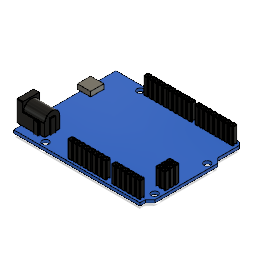
arduinoLeonardo (Autodesk Fusion 360 design; units mm, degrees)
Autodesk Fusion 360 part; units mm, degrees
note: some values were not read from the file. Chosen so that the rebuilt part matches the saved one: a direction; which face or edge a step refers to.
sketch "Sketch1" plane through (0, 0, 0) normal (0, 1, 0) x (1, 0, 0) in component "PCB"
  line L0 (0, 0) -> (64.5524, 0)
  line L1 (66.2, -1.6476) -> (66.2, -13)
  line L2 (66.2, -53.6) -> (0, -53.6)
  line L3 (0, -53.6) -> (0, 0)
  line L4 (64.5524, 0) -> (66.2, -1.6476)
  line L5 (64.5524, 0) -> (68.3345, 0) construction
  line L6 (64.5524, 0) -> (66.2, 0) construction
  line L7 (66.2, -13) -> (66.2, -50.8) construction
  line L8 (66.2, 0) -> (66.2, -1.6476) construction
  line L9 (66.2, -31.4728) -> (68.7, -31.4728) construction
  line L10 (66.2, -50.8) -> (66.2, -53.6)
  line L11 (66.2, -50.8) -> (68.7, -48.3)
  line L12 (66.2, -50.8) -> (70.1598, -50.8) construction
  line L13 (66.2, -13) -> (68.7, -15.5)
  line L14 (66.2, -13) -> (69.983, -13) construction
  line L15 (68.7, -15.5) -> (68.7, -48.3)
  dimension "d1" = 66.2
  dimension "d2" = 53.6
  dimension "d3" = 45
  dimension "d4" = 2.33
  dimension "d5" = 13
  dimension "d6" = 2.5
  dimension "d7" = 2.8
  dimension "d8" = 45
  dimension "d9" = 45
  dimension "d42" = 0
  dimension "d43" = 0
  dimension "d44" = 0
  dimension "d45" = 0
  dimension "d178" = 0
  dimension "d179" = 0
  dimension "d180" = 0
  dimension "d181" = 0
  measures "d3" angle of L4 L5
  measures "d8" angle of L11 L12
  measures "d9" angle of L13 L14
extrude "Extrude1" add sketch "Sketch1" along normal blind 1.62 makes body 1 in component "PCB"
sketch "Sketch1 (1)" plane through (0, 1.62, 0) normal (0, 1, 0) x (-1, 0, 0) in component "PCB"
  line L0 (-66.2, 50.8) -> (-68.7, 48.3)
  line L1 (-68.7, 48.3) -> (-68.7, 15.5)
  line L2 (-68.7, 15.5) -> (-66.2, 13)
  line L3 (-66.2, 13) -> (-66.2, 1.6476)
  line L4 (-66.2, 1.6476) -> (-64.5524, 0)
  line L5 (-64.5524, 0) -> (0, 0)
  line L6 (0, 0) -> (0, 53.6)
  line L7 (0, 53.6) -> (-66.2, 53.6)
  line L8 (-66.2, 53.6) -> (-66.2, 50.8)
  line L9 (-68.7, 31.9) -> (-67.7, 31.9) construction
  line L10 (-67.7, 18.15) -> (-67.7, 45.65) construction
  line L11 (-67.7, 18.15) -> (-65.95, 18.15) construction
  line L12 (-67.7, 45.65) -> (-65.95, 45.65) construction
  line L13 (-14, 53.6) -> (-14, 52.6) construction
  line L14 (-15.5, 0) -> (-15.5, 1) construction
  line L15 (-15.5, 1) -> (-15.5, 2.75) construction
  line L16 (-14, 52.6) -> (-14, 50.85) construction
  line L17 (0, 2.75) -> (-15.5, 2.75) construction
  line L18 (0, 50.85) -> (-14, 50.85) construction
  dimension "d12" = 1
  dimension "d13" = 27.5
  dimension "d14" = 1.75
  dimension "d15" = 1
  dimension "d16" = 1
  dimension "d17" = 1.75
  dimension "d18" = 1.75
  dimension "d19" = 15.5
  dimension "d20" = 14
  measures "d13" distance of L5.end
  measures "d20" distance of L5.end
hole "Hole1" at (15.5, 1.62, 2.75) at (14, 1.62, 50.85) at (65.95, 1.62, 45.65) at (65.95, 1.62, 18.15) direction (0, -1, 0) diameter 3.5 depth 1.62 tip angle 118 bodies 1 in component "PCB"
sketch "Sketch2" plane through (0, 1.62, 0) normal (0, 1, 0) x (-1, 0, 0) in component "PCB"
  circle A0 centre (-65.95, 45.65) radius 1.75
  circle A1 centre (-15.5, 2.75) radius 1.75
  circle A2 centre (-14, 50.85) radius 1.75
  circle A3 centre (-65.95, 18.15) radius 1.75
  line L0 (-66.2, 50.8) -> (-68.7, 48.3)
  line L1 (-68.7, 48.3) -> (-68.7, 15.5)
  line L2 (-68.7, 15.5) -> (-66.2, 13)
  line L3 (-66.2, 13) -> (-66.2, 1.6476)
  line L4 (-66.2, 1.6476) -> (-64.5524, 0)
  line L5 (-64.5524, 0) -> (0, 0)
  line L6 (0, 0) -> (0, 53.6)
  line L7 (0, 53.6) -> (-66.2, 53.6)
  line L8 (-66.2, 53.6) -> (-66.2, 50.8)
  line L9 (-64.3788, 0) -> (-64.3788, 2.5) construction
  line L10 (-65.4815, 53.6) -> (-65.4815, 51.1) construction
  line L11 (-66.2, 2.5) -> (-63.7, 2.5) construction
  line L12 (-66.2, 51.1) -> (-63.7, 51.1) construction
  line L13 (-63.7, 51.1) -> (-61.16, 51.1) construction
  line L14 (-61.16, 51.1) -> (-58.62, 51.1) construction
  line L15 (-58.62, 51.1) -> (-56.08, 51.1) construction
  line L16 (-56.08, 51.1) -> (-53.54, 51.1) construction
  line L17 (-53.54, 51.1) -> (-51, 51.1) construction
  line L18 (-51, 51.1) -> (-46, 51.1) construction
  line L19 (-46, 51.1) -> (-43.46, 51.1) construction
  line L20 (-43.46, 51.1) -> (-40.92, 51.1) construction
  line L21 (-40.92, 51.1) -> (-38.38, 51.1) construction
  line L22 (-38.38, 51.1) -> (-35.84, 51.1) construction
  line L23 (-35.84, 51.1) -> (-33.3, 51.1) construction
  line L24 (-33.3, 51.1) -> (-30.76, 51.1) construction
  line L25 (-30.76, 51.1) -> (-28.22, 51.1) construction
  line L26 (-28.22, 51.1) -> (-25.68, 51.1) construction
  line L27 (-63.7, 2.5) -> (-61.16, 2.5) construction
  line L28 (-61.16, 2.5) -> (-58.62, 2.5) construction
  line L29 (-58.62, 2.5) -> (-56.08, 2.5) construction
  line L30 (-56.08, 2.5) -> (-53.54, 2.5) construction
  line L31 (-53.54, 2.5) -> (-51, 2.5) construction
  line L32 (-51, 2.5) -> (-48.46, 2.5) construction
  line L33 (-45.92, 2.5114) -> (-48.46, 2.5) construction
  line L34 (-45.92, 2.5114) -> (-42.1201, 2.5284) construction
  line L35 (-42.1201, 2.5284) -> (-39.5801, 2.5398) construction
  line L36 (-39.5801, 2.5398) -> (-37.0401, 2.5511) construction
  line L37 (-37.0401, 2.5511) -> (-34.5001, 2.5625) construction
  line L38 (-34.5001, 2.5625) -> (-31.9602, 2.5739) construction
  line L39 (-31.9602, 2.5739) -> (-29.4202, 2.5853) construction
  line L40 (-29.4202, 2.5853) -> (-26.8802, 2.5966) construction
  line L41 (-26.8802, 2.5966) -> (-24.3402, 2.608) construction
  line L42 (-24.3402, 2.608) -> (-21.8003, 2.6194) construction
  line L43 (-21.8003, 2.6194) -> (-19.2603, 2.6307) construction
  line L44 (-68.7, 40.6001) -> (-66.2, 40.6001) construction
  line L45 (-65.9335, 43.9001) -> (-65.9335, 40.6001) construction
  line L46 (-66.2, 40.6001) -> (-66.2, 38.0601) construction
  line L47 (-66.2, 38.0601) -> (-66.2, 35.5201) construction
  line L48 (-66.2, 35.5201) -> (-63.66, 35.5201) construction
  line L49 (-63.66, 35.5201) -> (-63.66, 38.0601) construction
  line L50 (-63.66, 38.0601) -> (-63.66, 40.6001) construction
  dimension "d24" = 2.5
  dimension "d25" = 2.5
  dimension "d26" = 2.5
  dimension "d27" = 2.5
  dimension "d28" = 2.54
  dimension "d29" = 5
  dimension "d30" = 2.54
  dimension "d31" = 3.8
  dimension "d32" = 2.5
  dimension "d33" = 3.3
  dimension "d34" = 2.54
  measures "d24" distance of L5.end
hole "Hole2" at (63.7, 1.62, 51.1) at (61.16, 1.62, 51.1) at (58.62, 1.62, 51.1) at (56.08, 1.62, 51.1) at (53.54, 1.62, 51.1) at (51, 1.62, 51.1) at (46, 1.62, 51.1) at (43.46, 1.62, 51.1) at (40.92, 1.62, 51.1) at (38.38, 1.62, 51.1) at (35.84, 1.62, 51.1) at (33.3, 1.62, 51.1) at (30.76, 1.62, 51.1) at (28.22, 1.62, 51.1) at (63.66, 1.62, 40.6001) at (63.66, 1.62, 38.0601) at (63.66, 1.62, 35.5201) at (66.2, 1.62, 35.5201) at (66.2, 1.62, 38.0601) at (66.2, 1.62, 40.6001) at (63.7, 1.62, 2.5) at (61.16, 1.62, 2.5) at (58.62, 1.62, 2.5) at (56.08, 1.62, 2.5) at (53.54, 1.62, 2.5) at (51, 1.62, 2.5) at (48.46, 1.62, 2.5) at (45.92, 1.62, 2.5114) at (42.1201, 1.62, 2.5284) at (39.5801, 1.62, 2.5398) at (37.0401, 1.62, 2.5511) at (34.5001, 1.62, 2.5625) at (31.9602, 1.62, 2.5739) at (29.4202, 1.62, 2.5853) at (26.8802, 1.62, 2.5966) at (24.3402, 1.62, 2.608) at (21.8003, 1.62, 2.6194) at (19.2603, 1.62, 2.6307) direction (0, -1, 0) diameter 0.635 depth 1.62 tip angle 118 bodies 1 in component "PCB"
sketch "Sketch1 (2)" plane through (0, 0, 0) normal (0, 1, 0) x (1, 0, 0) in component "Pin"
  line L0 (0, 0) -> (5.08, 0)
  line L1 (5.08, 0) -> (5.08, -0.635)
  line L2 (5.08, -0.635) -> (0, -0.635)
  line L3 (0, -0.635) -> (0, 0)
  dimension "d2_1" = 0.635
  dimension "d3_1" = 5.08
  measures "d3_1" distance of L0.start
extrude "Extrude1'" add sketch "Sketch1 (2)" along normal blind 0.635 separate body makes body 2 in component "Pin"
chamfer "Chamfer1" distance 0.1905 angle 45 4 edges at (0, 0.3175, 0.635) (0, 0.635, 0.3175) (0, 0.3175, 0) (0, 0, 0.3175) on bodies 2 in component "Pin"
sketch "Sketch1 (3)" plane through (0, 0, 0) normal (0, 1, 0) x (1, 0, 0) in component "Plastic"
  line L0 (0, -0.3175) -> (3.81, -0.3175)
  line L1 (3.81, -1.0795) -> (3.81, 0.4445)
  line L2 (3.81, 0.4445) -> (3.8102, 0.9525) construction
  line L3 (3.81, -1.0795) -> (3.81, -1.5875) construction
  line L4 (3.81, 0.4445) -> (3.175, 0.4445)
  line L5 (3.81, -1.0795) -> (3.175, -1.0795)
  line L6 (3.175, -1.0795) -> (3.175, -1.5875)
  line L7 (3.175, 0.4445) -> (3.175, 0.9525)
  line L8 (3.175, 0.9525) -> (11.811, 0.9525)
  line L9 (11.811, 0.9525) -> (11.811, -1.5875)
  line L10 (3.175, -1.5875) -> (11.811, -1.5875)
  line L11 (0, -0.1905) -> (0, -0.4445)
  dimension "d7_1" = 3.81
  dimension "d8_1" = 1.524
  dimension "d9_1" = 0.508
  dimension "d11_1" = 0.635
  dimension "d12_1" = 8.636
  measures "d7_1" distance of origin
extrude "Extrude1''" add sketch "Sketch1 (3)" along normal mid plane 2.54 from surface at 0.3175 separate body makes body 3 in component "Plastic"
chamfer "Chamfer1'" distance 0.4 angle 45 4 edges at (7.493, 1.5875, -0.9525) (7.493, -0.9525, -0.9525) (7.493, 1.5875, 1.5875) (7.493, -0.9525, 1.5875) on bodies 3 in component "Plastic"
sketch "Sketch1 (4)" plane through (0, 0, 0) normal (0, 0, 1) x (1, 0, 0) in component "Pins straight female v5"
  line L0 (0, 0.1905) -> (0, 0.4445)
  line L1 (0, 0.3175) -> (0, 14)
other "PathPattern1" in component "Header"
sketch "Sketch1 (1) (2)" plane through (11.811, 0, 0) normal (1, 0, 0) x (0, 0, -1) in component "Plastic"
  line L0 (-1.5875, -0.5525) -> (-1.1875, -0.9525)
  line L1 (-1.1875, -0.9525) -> (0.5525, -0.9525)
  line L2 (0.5525, -0.9525) -> (0.9525, -0.5525)
  line L3 (0.9525, -0.5525) -> (0.9525, 1.1875)
  line L4 (0.9525, 1.1875) -> (0.5525, 1.5875)
  line L5 (0.5525, 1.5875) -> (-1.1875, 1.5875)
  line L6 (-1.1875, 1.5875) -> (-1.5875, 1.1875)
  line L7 (-1.5875, 1.1875) -> (-1.5875, -0.5525)
  line L8 (0.9525, 0.3175) -> (-0.3175, 0.3175) construction
  line L9 (-0.3175, 1.5875) -> (-0.3175, 0.3175) construction
  line L10 (-0.3175, 0.635) -> (0, 0.635)
  line L11 (0, 0.3175) -> (0, 0)
  line L12 (0, 0) -> (-0.635, 0)
  line L13 (-0.635, 0) -> (-0.635, 0.635)
  line L14 (0, 0.635) -> (0, 0.3175)
  line L15 (-0.635, 0.635) -> (-0.3175, 0.635)
  dimension "d24_1" = 0.635
  dimension "d25_1" = 0.635
  measures "d25_1" distance of L11.end
extrude "Extrude1'''" cut sketch "Sketch1 (1) (2)" against normal blind 5.5 contours L10 L11 L12 L13 L14 L15 bodies 3 in component "Plastic"
chamfer "Chamfer1''" distance 0.6 angle 45 4 edges at (11.811, 0, 0.3175) (11.811, 0.3175, 0) (11.811, 0.635, 0.3175) (11.811, 0.3175, 0.635) on bodies 3 in component "Plastic"
sketch "Sketch1 (5)" plane through (0, 0, 0) normal (0, 1, 0) x (1, 0, 0) in component "Pin (1)"
  line L0 (0, 0) -> (5.08, 0)
  line L1 (5.08, 0) -> (5.08, -0.635)
  line L2 (5.08, -0.635) -> (0, -0.635)
  line L3 (0, -0.635) -> (0, 0)
  dimension "d2_2" = 0.635
  dimension "d3_2" = 5.08
  measures "d3_2" distance of L0.start
extrude "Extrude1''''" add sketch "Sketch1 (5)" along normal blind 0.635 separate body makes body 4 in component "Pin (1)"
chamfer "Chamfer1'''" distance 0.1905 angle 45 4 edges at (0, 0.3175, 0.635) (0, 0.635, 0.3175) (0, 0.3175, 0) (0, 0, 0.3175) on bodies 4 in component "Pin (1)"
sketch "Sketch1 (6)" plane through (0, 0, 0) normal (0, 1, 0) x (1, 0, 0) in component "Plastic (1)"
  line L0 (0, -0.3175) -> (3.81, -0.3175)
  line L1 (3.81, -1.0795) -> (3.81, 0.4445)
  line L2 (3.81, 0.4445) -> (3.8102, 0.9525) construction
  line L3 (3.81, -1.0795) -> (3.81, -1.5875) construction
  line L4 (3.81, 0.4445) -> (3.175, 0.4445)
  line L5 (3.81, -1.0795) -> (3.175, -1.0795)
  line L6 (3.175, -1.0795) -> (3.175, -1.5875)
  line L7 (3.175, 0.4445) -> (3.175, 0.9525)
  line L8 (3.175, 0.9525) -> (11.811, 0.9525)
  line L9 (11.811, 0.9525) -> (11.811, -1.5875)
  line L10 (3.175, -1.5875) -> (11.811, -1.5875)
  line L11 (0, -0.1905) -> (0, -0.4445)
  dimension "d7_2" = 3.81
  dimension "d8_2" = 1.524
  dimension "d9_2" = 0.508
  dimension "d11_2" = 0.635
  dimension "d12_2" = 8.636
  measures "d7_2" distance of origin
extrude "Extrude1'''''" add sketch "Sketch1 (6)" along normal mid plane 2.54 from surface at 0.3175 separate body makes body 5 in component "Plastic (1)"
chamfer "Chamfer1''''" distance 0.4 angle 45 4 edges at (7.493, 1.5875, -0.9525) (7.493, -0.9525, -0.9525) (7.493, 1.5875, 1.5875) (7.493, -0.9525, 1.5875) on bodies 5 in component "Plastic (1)"
sketch "Sketch1 (7)" plane through (0, 0, 0) normal (0, 0, 1) x (1, 0, 0) in component "Pins straight female v6"
  line L0 (0, 0.1905) -> (0, 0.4445)
  line L1 (0, 0.3175) -> (0, 14)
other "PathPattern1'" in component "Header (1)"
sketch "Sketch1 (1) (3)" plane through (11.811, 0, 0) normal (1, 0, 0) x (0, 0, -1) in component "Plastic (1)"
  line L0 (-1.5875, -0.5525) -> (-1.1875, -0.9525)
  line L1 (-1.1875, -0.9525) -> (0.5525, -0.9525)
  line L2 (0.5525, -0.9525) -> (0.9525, -0.5525)
  line L3 (0.9525, -0.5525) -> (0.9525, 1.1875)
  line L4 (0.9525, 1.1875) -> (0.5525, 1.5875)
  line L5 (0.5525, 1.5875) -> (-1.1875, 1.5875)
  line L6 (-1.1875, 1.5875) -> (-1.5875, 1.1875)
  line L7 (-1.5875, 1.1875) -> (-1.5875, -0.5525)
  line L8 (0.9525, 0.3175) -> (-0.3175, 0.3175) construction
  line L9 (-0.3175, 1.5875) -> (-0.3175, 0.3175) construction
  line L10 (-0.3175, 0.635) -> (0, 0.635)
  line L11 (0, 0.3175) -> (0, 0)
  line L12 (0, 0) -> (-0.635, 0)
  line L13 (-0.635, 0) -> (-0.635, 0.635)
  line L14 (0, 0.635) -> (0, 0.3175)
  line L15 (-0.635, 0.635) -> (-0.3175, 0.635)
  dimension "d24_2" = 0.635
  dimension "d25_2" = 0.635
  measures "d25_2" distance of L11.end
extrude "Extrude1''''''" cut sketch "Sketch1 (1) (3)" against normal blind 5.5 contours L10 L11 L12 L13 L14 L15 bodies 5 in component "Plastic (1)"
chamfer "Chamfer1'''''" distance 0.6 angle 45 4 edges at (11.811, 0, 0.3175) (11.811, 0.3175, 0) (11.811, 0.635, 0.3175) (11.811, 0.3175, 0.635) on bodies 5 in component "Plastic (1)"
sketch "Sketch1 (8)" plane through (0, 0, 0) normal (0, 1, 0) x (1, 0, 0) in component "Pin (2)"
  line L0 (0, 0) -> (5.08, 0)
  line L1 (5.08, 0) -> (5.08, -0.635)
  line L2 (5.08, -0.635) -> (0, -0.635)
  line L3 (0, -0.635) -> (0, 0)
  dimension "d2_3" = 0.635
  dimension "d3_3" = 5.08
  dimension "d38" = 0
  dimension "d39" = 0
  dimension "d40" = 0
  dimension "d41" = 0
  measures "d3_3" distance of L0.start
extrude "Extrude1'''''''" add sketch "Sketch1 (8)" along normal blind 0.635 separate body makes body 6 in component "Pin (2)"
chamfer "Chamfer1''''''" distance 0.1905 angle 45 4 edges at (0, 0.3175, 0.635) (0, 0.635, 0.3175) (0, 0.3175, 0) (0, 0, 0.3175) on bodies 6 in component "Pin (2)"
sketch "Sketch1 (9)" plane through (0, 0, 0) normal (0, 1, 0) x (1, 0, 0) in component "Plastic (2)"
  line L0 (0, -0.3175) -> (3.81, -0.3175)
  line L1 (3.81, -1.0795) -> (3.81, 0.4445)
  line L2 (3.81, 0.4445) -> (3.8102, 0.9525) construction
  line L3 (3.81, -1.0795) -> (3.81, -1.5875) construction
  line L4 (3.81, 0.4445) -> (3.175, 0.4445)
  line L5 (3.81, -1.0795) -> (3.175, -1.0795)
  line L6 (3.175, -1.0795) -> (3.175, -1.5875)
  line L7 (3.175, 0.4445) -> (3.175, 0.9525)
  line L8 (3.175, 0.9525) -> (11.811, 0.9525)
  line L9 (11.811, 0.9525) -> (11.811, -1.5875)
  line L10 (3.175, -1.5875) -> (11.811, -1.5875)
  line L11 (0, -0.1905) -> (0, -0.4445)
  dimension "d7_3" = 3.81
  dimension "d8_3" = 1.524
  dimension "d9_3" = 0.508
  dimension "d11_3" = 0.635
  dimension "d12_3" = 8.636
  measures "d7_3" distance of origin
extrude "Extrude1''''''''" add sketch "Sketch1 (9)" along normal mid plane 2.54 from surface at 0.3175 separate body makes body 7 in component "Plastic (2)"
chamfer "Chamfer1'''''''" distance 0.4 angle 45 4 edges at (7.493, 1.5875, -0.9525) (7.493, -0.9525, -0.9525) (7.493, 1.5875, 1.5875) (7.493, -0.9525, 1.5875) on bodies 7 in component "Plastic (2)"
sketch "Sketch1 (10)" plane through (0, 0, 0) normal (0, 0, 1) x (1, 0, 0) in component "Pins straight female v7"
  line L0 (0, 0.1905) -> (0, 0.4445)
  line L1 (0, 0.3175) -> (0, 14)
other "PathPattern1''" in component "Header (2)"
sketch "Sketch1 (1) (4)" plane through (11.811, 0, 0) normal (1, 0, 0) x (0, 0, -1) in component "Plastic (2)"
  line L0 (-1.5875, -0.5525) -> (-1.1875, -0.9525)
  line L1 (-1.1875, -0.9525) -> (0.5525, -0.9525)
  line L2 (0.5525, -0.9525) -> (0.9525, -0.5525)
  line L3 (0.9525, -0.5525) -> (0.9525, 1.1875)
  line L4 (0.9525, 1.1875) -> (0.5525, 1.5875)
  line L5 (0.5525, 1.5875) -> (-1.1875, 1.5875)
  line L6 (-1.1875, 1.5875) -> (-1.5875, 1.1875)
  line L7 (-1.5875, 1.1875) -> (-1.5875, -0.5525)
  line L8 (0.9525, 0.3175) -> (-0.3175, 0.3175) construction
  line L9 (-0.3175, 1.5875) -> (-0.3175, 0.3175) construction
  line L10 (-0.3175, 0.635) -> (0, 0.635)
  line L11 (0, 0.3175) -> (0, 0)
  line L12 (0, 0) -> (-0.635, 0)
  line L13 (-0.635, 0) -> (-0.635, 0.635)
  line L14 (0, 0.635) -> (0, 0.3175)
  line L15 (-0.635, 0.635) -> (-0.3175, 0.635)
  dimension "d24_3" = 0.635
  dimension "d25_3" = 0.635
  measures "d25_3" distance of L11.end
extrude "Extrude1'''''''''" cut sketch "Sketch1 (1) (4)" against normal blind 5.5 contours L10 L11 L12 L13 L14 L15 bodies 7 in component "Plastic (2)"
chamfer "Chamfer1''''''''" distance 0.6 angle 45 4 edges at (11.811, 0, 0.3175) (11.811, 0.3175, 0) (11.811, 0.635, 0.3175) (11.811, 0.3175, 0.635) on bodies 7 in component "Plastic (2)"
sketch "Sketch1 (11)" plane through (0, 0, 0) normal (0, 1, 0) x (1, 0, 0) in component "Pin (3)"
  line L0 (0, 0) -> (5.08, 0)
  line L1 (5.08, 0) -> (5.08, -0.635)
  line L2 (5.08, -0.635) -> (0, -0.635)
  line L3 (0, -0.635) -> (0, 0)
  dimension "d2_4" = 0.635
  dimension "d3_4" = 5.08
  measures "d3_4" distance of L0.start
extrude "Extrude1''''''''''" add sketch "Sketch1 (11)" along normal blind 0.635 separate body makes body 8 in component "Pin (3)"
chamfer "Chamfer1'''''''''" distance 0.1905 angle 45 4 edges at (0, 0.3175, 0.635) (0, 0.635, 0.3175) (0, 0.3175, 0) (0, 0, 0.3175) on bodies 8 in component "Pin (3)"
sketch "Sketch1 (12)" plane through (0, 0, 0) normal (0, 1, 0) x (1, 0, 0) in component "Plastic (3)"
  line L0 (0, -0.3175) -> (3.81, -0.3175)
  line L1 (3.81, -1.0795) -> (3.81, 0.4445)
  line L2 (3.81, 0.4445) -> (3.8102, 0.9525) construction
  line L3 (3.81, -1.0795) -> (3.81, -1.5875) construction
  line L4 (3.81, 0.4445) -> (3.175, 0.4445)
  line L5 (3.81, -1.0795) -> (3.175, -1.0795)
  line L6 (3.175, -1.0795) -> (3.175, -1.5875)
  line L7 (3.175, 0.4445) -> (3.175, 0.9525)
  line L8 (3.175, 0.9525) -> (11.811, 0.9525)
  line L9 (11.811, 0.9525) -> (11.811, -1.5875)
  line L10 (3.175, -1.5875) -> (11.811, -1.5875)
  line L11 (0, -0.1905) -> (0, -0.4445)
  dimension "d7_4" = 3.81
  dimension "d8_4" = 1.524
  dimension "d9_4" = 0.508
  dimension "d11_4" = 0.635
  dimension "d12_4" = 8.636
  measures "d7_4" distance of origin
extrude "Extrude1'''''''''''" add sketch "Sketch1 (12)" along normal mid plane 2.54 from surface at 0.3175 separate body makes body 9 in component "Plastic (3)"
chamfer "Chamfer1''''''''''" distance 0.4 angle 45 4 edges at (7.493, 1.5875, -0.9525) (7.493, -0.9525, -0.9525) (7.493, 1.5875, 1.5875) (7.493, -0.9525, 1.5875) on bodies 9 in component "Plastic (3)"
sketch "Sketch1 (13)" plane through (0, 0, 0) normal (0, 0, 1) x (1, 0, 0) in component "Pins straight female v8"
  line L0 (0, 0.1905) -> (0, 0.4445)
  line L1 (0, 0.3175) -> (0, 14)
other "PathPattern1'''" in component "Header (3)"
sketch "Sketch1 (1) (5)" plane through (11.811, 0, 0) normal (1, 0, 0) x (0, 0, -1) in component "Plastic (3)"
  line L0 (-1.5875, -0.5525) -> (-1.1875, -0.9525)
  line L1 (-1.1875, -0.9525) -> (0.5525, -0.9525)
  line L2 (0.5525, -0.9525) -> (0.9525, -0.5525)
  line L3 (0.9525, -0.5525) -> (0.9525, 1.1875)
  line L4 (0.9525, 1.1875) -> (0.5525, 1.5875)
  line L5 (0.5525, 1.5875) -> (-1.1875, 1.5875)
  line L6 (-1.1875, 1.5875) -> (-1.5875, 1.1875)
  line L7 (-1.5875, 1.1875) -> (-1.5875, -0.5525)
  line L8 (0.9525, 0.3175) -> (-0.3175, 0.3175) construction
  line L9 (-0.3175, 1.5875) -> (-0.3175, 0.3175) construction
  line L10 (-0.3175, 0.635) -> (0, 0.635)
  line L11 (0, 0.3175) -> (0, 0)
  line L12 (0, 0) -> (-0.635, 0)
  line L13 (-0.635, 0) -> (-0.635, 0.635)
  line L14 (0, 0.635) -> (0, 0.3175)
  line L15 (-0.635, 0.635) -> (-0.3175, 0.635)
  dimension "d24_4" = 0.635
  dimension "d25_4" = 0.635
  measures "d25_4" distance of L11.end
extrude "Extrude1''''''''''''" cut sketch "Sketch1 (1) (5)" against normal blind 5.5 contours L10 L11 L12 L13 L14 L15 bodies 9 in component "Plastic (3)"
chamfer "Chamfer1'''''''''''" distance 0.6 angle 45 4 edges at (11.811, 0, 0.3175) (11.811, 0.3175, 0) (11.811, 0.635, 0.3175) (11.811, 0.3175, 0.635) on bodies 9 in component "Plastic (3)"
sketch "Sketch3" plane through (0, 1.62, 0) normal (0, 1, 0) x (-1, 0, 0) in component "PCB"
  circle A0 centre (-21.8003, 2.6194) radius 0.3175
  circle A1 centre (-26.8802, 2.5966) radius 0.3175
  circle A2 centre (-31.9602, 2.5739) radius 0.3175
  circle A3 centre (-37.0401, 2.5511) radius 0.3175
  circle A4 centre (-42.1201, 2.5284) radius 0.3175
  circle A5 centre (-48.46, 2.5) radius 0.3175
  circle A6 centre (-53.54, 2.5) radius 0.3175
  circle A7 centre (-58.62, 2.5) radius 0.3175
  circle A8 centre (-63.7, 2.5) radius 0.3175
  circle A9 centre (-66.2, 38.0601) radius 0.3175
  circle A10 centre (-63.66, 35.5201) radius 0.3175
  circle A11 centre (-63.66, 40.6001) radius 0.3175
  circle A12 centre (-30.76, 51.1) radius 0.3175
  circle A13 centre (-35.84, 51.1) radius 0.3175
  circle A14 centre (-40.92, 51.1) radius 0.3175
  circle A15 centre (-46, 51.1) radius 0.3175
  circle A16 centre (-53.54, 51.1) radius 0.3175
  circle A17 centre (-58.62, 51.1) radius 0.3175
  circle A18 centre (-63.7, 51.1) radius 0.3175
  circle A19 centre (-61.16, 51.1) radius 0.3175
  circle A20 centre (-56.08, 51.1) radius 0.3175
  circle A21 centre (-51, 51.1) radius 0.3175
  circle A22 centre (-43.46, 51.1) radius 0.3175
  circle A23 centre (-38.38, 51.1) radius 0.3175
  circle A24 centre (-33.3, 51.1) radius 0.3175
  circle A25 centre (-28.22, 51.1) radius 0.3175
  circle A26 centre (-63.66, 38.0601) radius 0.3175
  circle A27 centre (-66.2, 35.5201) radius 0.3175
  circle A28 centre (-66.2, 40.6001) radius 0.3175
  circle A29 centre (-61.16, 2.5) radius 0.3175
  circle A30 centre (-56.08, 2.5) radius 0.3175
  circle A31 centre (-51, 2.5) radius 0.3175
  circle A32 centre (-45.92, 2.5114) radius 0.3175
  circle A33 centre (-39.5801, 2.5398) radius 0.3175
  circle A34 centre (-34.5001, 2.5625) radius 0.3175
  circle A35 centre (-29.4202, 2.5853) radius 0.3175
  circle A36 centre (-24.3402, 2.608) radius 0.3175
  circle A37 centre (-19.2603, 2.6307) radius 0.3175
  circle A38 centre (-65.95, 45.65) radius 1.75
  circle A39 centre (-15.5, 2.75) radius 1.75
  circle A40 centre (-14, 50.85) radius 1.75
  circle A41 centre (-65.95, 18.15) radius 1.75
  line L0 (-66.2, 50.8) -> (-68.7, 48.3)
  line L1 (-68.7, 48.3) -> (-68.7, 15.5)
  line L2 (-68.7, 15.5) -> (-66.2, 13)
  line L3 (-66.2, 13) -> (-66.2, 1.6476)
  line L4 (-66.2, 1.6476) -> (-64.5524, 0)
  line L5 (-64.5524, 0) -> (0, 0)
  line L6 (0, 0) -> (0, 53.6)
  line L7 (0, 53.6) -> (-66.2, 53.6)
  line L8 (-66.2, 53.6) -> (-66.2, 50.8)
  line L9 (-4, 0) -> (-4, 15) construction
  line L10 (0, 15) -> (-4, 15) construction
  line L11 (-4, 12.575) -> (-4, 17.425) construction
  dimension "d118" = 15
  dimension "d119" = 4
  dimension "d120" = 4.85
hole "Hole3" at (4, 1.62, 12.575) at (4, 1.62, 17.425) direction (0, -1, 0) diameter 0.635 depth 1.62 tip angle 118 bodies 1 in component "PCB"
sketch "Sketch1 (14)" plane through (0, 1.62, 0) normal (0, 1, 0) x (-1, 0, 0) in component "PCB"
  circle A0 centre (-4, 12.575) radius 0.3175
  circle A1 centre (-4, 17.425) radius 0.3175
  circle A2 centre (-21.8003, 2.6194) radius 0.3175
  circle A3 centre (-26.8802, 2.5966) radius 0.3175
  circle A4 centre (-31.9602, 2.5739) radius 0.3175
  circle A5 centre (-37.0401, 2.5511) radius 0.3175
  circle A6 centre (-42.1201, 2.5284) radius 0.3175
  circle A7 centre (-48.46, 2.5) radius 0.3175
  circle A8 centre (-53.54, 2.5) radius 0.3175
  circle A9 centre (-58.62, 2.5) radius 0.3175
  circle A10 centre (-63.7, 2.5) radius 0.3175
  circle A11 centre (-66.2, 38.0601) radius 0.3175
  circle A12 centre (-63.66, 35.5201) radius 0.3175
  circle A13 centre (-63.66, 40.6001) radius 0.3175
  circle A14 centre (-30.76, 51.1) radius 0.3175
  circle A15 centre (-35.84, 51.1) radius 0.3175
  circle A16 centre (-40.92, 51.1) radius 0.3175
  circle A17 centre (-46, 51.1) radius 0.3175
  circle A18 centre (-53.54, 51.1) radius 0.3175
  circle A19 centre (-58.62, 51.1) radius 0.3175
  circle A20 centre (-63.7, 51.1) radius 0.3175
  circle A21 centre (-61.16, 51.1) radius 0.3175
  circle A22 centre (-56.08, 51.1) radius 0.3175
  circle A23 centre (-51, 51.1) radius 0.3175
  circle A24 centre (-43.46, 51.1) radius 0.3175
  circle A25 centre (-38.38, 51.1) radius 0.3175
  circle A26 centre (-33.3, 51.1) radius 0.3175
  circle A27 centre (-28.22, 51.1) radius 0.3175
  circle A28 centre (-63.66, 38.0601) radius 0.3175
  circle A29 centre (-66.2, 35.5201) radius 0.3175
  circle A30 centre (-66.2, 40.6001) radius 0.3175
  circle A31 centre (-61.16, 2.5) radius 0.3175
  circle A32 centre (-56.08, 2.5) radius 0.3175
  circle A33 centre (-51, 2.5) radius 0.3175
  circle A34 centre (-45.92, 2.5114) radius 0.3175
  circle A35 centre (-39.5801, 2.5398) radius 0.3175
  circle A36 centre (-34.5001, 2.5625) radius 0.3175
  circle A37 centre (-29.4202, 2.5853) radius 0.3175
  circle A38 centre (-24.3402, 2.608) radius 0.3175
  circle A39 centre (-19.2603, 2.6307) radius 0.3175
  circle A40 centre (-65.95, 45.65) radius 1.75
  circle A41 centre (-15.5, 2.75) radius 1.75
  circle A42 centre (-14, 50.85) radius 1.75
  circle A43 centre (-65.95, 18.15) radius 1.75
  line L0 (-66.2, 50.8) -> (-68.7, 48.3)
  line L1 (-68.7, 48.3) -> (-68.7, 15.5)
  line L2 (-68.7, 15.5) -> (-66.2, 13)
  line L3 (-66.2, 13) -> (-66.2, 1.6476)
  line L4 (-66.2, 1.6476) -> (-64.5524, 0)
  line L5 (-64.5524, 0) -> (0, 0)
  line L6 (0, 0) -> (0, 53.6)
  line L7 (0, 53.6) -> (-66.2, 53.6)
  line L8 (-66.2, 53.6) -> (-66.2, 50.8)
  line L9 (0, 45.1) -> (-12, 45.1) construction
  line L10 (-12, 45.1) -> (-12, 53.6) construction
  dimension "d136" = 12
  dimension "d137" = 8.5
  measures "d136" distance of L5.end
sketch "Sketch1 (15)" plane through (0, 0, 0) normal (0, 1, 0) x (1, 0, 0) in component "DC Jack"
  line L0 (0, 0) -> (9, 0)
  line L1 (9, 0) -> (9, -11)
  line L2 (9, -11) -> (0, -11)
  line L3 (0, -11) -> (0, 0)
  dimension "d1_1" = 9
  dimension "d2_5" = 11
  measures "d1_1" distance of L0.start
  measures "d2_5" distance of L0.start
extrude "Extrude1'''''''''''''" add sketch "Sketch1 (15)" along normal blind 3.3 separate body makes body 10 in component "DC Jack"
sketch "Sketch2 (2)" plane through (0, 3.3, 0) normal (0, 1, 0) x (-1, 0, 0) in component "DC Jack"
  line L0 (0, 11) -> (-9, 11)
  line L1 (-9, 11) -> (-9, 0)
  line L2 (-9, 0) -> (0, 0)
  line L3 (0, 0) -> (0, 11)
  circle A0 centre (-4.5, 4.75) radius 3.95
  line L4 (-4.5, 0) -> (-4.5, 0.8) construction
  line L5 (-9, 4.75) -> (-8.45, 4.75)
  line L6 (0, 4.75) -> (-0.55, 4.75)
  dimension "d5_5" = 0.8
  dimension "d6_5" = 7.9
  measures "d6_5" diameter of A0
extrude "Extrude2" add sketch "Sketch2 (2)" along normal blind 8.5 contours L0 L1 L3 A0 L5 L6 | A0 bodies 10 in component "DC Jack"
sketch "Sketch3 (2)" plane through (0, 11.8, 0) normal (0, 1, 0) x (-1, 0, 0) in component "DC Jack"
  line L0 (0, 11) -> (-9, 11)
  line L1 (-9, 11) -> (-9, 4.75)
  line L2 (-9, 4.75) -> (-8.45, 4.75)
  arc A0 (-8.45, 4.75) -> (-0.55, 4.75) centre (-4.5, 4.75) ccw
  line L3 (-0.55, 4.75) -> (0, 4.75)
  line L4 (0, 4.75) -> (0, 11)
  line L5 (-0.55, 4.75) -> (-0.55, 11)
  line L6 (-8.45, 4.75) -> (-8.45, 11)
extrude "Extrude3" add sketch "Sketch3 (2)" along normal blind 2.4 contours L0 A0 L5 L6 bodies 10 in component "DC Jack"
sketch "Sketch4" plane through (0, 0, 0) normal (0, -1, 0) x (1, 0, 0) in component "DC Jack"
  line L0 (9, 11) -> (0, 11)
  line L1 (0, 11) -> (0, 0)
  line L2 (0, 0) -> (9, 0)
  line L3 (9, 0) -> (9, 11)
hole "Hole1'" at (4.5, 0, 4.75) direction (0, 1, 0) diameter 6.5 depth 9.6 tip angle 180 bodies 10 in component "DC Jack"
sketch "Sketch1 (16)" plane through (0, 9.6, 0) normal (0, -1, 0) x (1, 0, 0) in component "Connection"
  circle A0 centre (4.5, 4.75) radius 3.25
  circle A1 centre (4.5, 4.75) radius 1.25
  dimension "d14_5" = 2.5
  measures "d14_5" diameter of A1
extrude "Extrude1''''''''''''''" add sketch "Sketch1 (16)" along normal blind 8.1 separate body contours A1 makes body 11 in component "Connection"
ref_plane "WorkPlane1" through (1.2501, 0.7141, 4.7724) normal (0.999976, 0, -0.006903) x (0.006903, 0, 0.999976) in component "Connection"
ref_plane "WorkPlane2" through (3.2501, 2.383, 4.7654) normal (-0.999924, 0, 0.012358) x (0.012358, 0, 0.999924) in component "Connection"
ref_plane "WorkPlane3" through (2.2501, 2.383, 4.7764) normal (-0.999954, 0, 0.009631) x (0.009631, 0, 0.999954) in component "Connection"
sketch "Sketch2 (3)" plane through (2.2501, 2.383, 4.7764) normal (-0.999954, 0, 0.009631) x (0.009631, 0, 0.999954) in component "Connection"
  line L0 (0.0386, 0.917) -> (-4.7112, 0.917)
  line L1 (-2.5152, 0.917) -> (-2.5152, 2.9)
  line L2 (-2.5152, 2.9) -> (-1.4, 4.1)
  line L3 (-1.4, 4.1) -> (-2.5152, 5.8045)
  line L4 (-2.5152, 5.8045) -> (-2.6321, 5.728)
  line L5 (-2.6321, 5.728) -> (-1.567, 4.1)
  line L6 (-1.567, 4.1) -> (-2.6321, 2.9477)
  line L7 (-2.6321, 2.9477) -> (-2.6321, 0.917)
extrude "Extrude2'" add sketch "Sketch2 (3)" against normal blind 4.54 separate body makes body 12 in component "Connection"
move_body "Move1" bodies 12 to x (1, 0, 0) y (0, -1, 0) z (0, 0, -1) at (0.0109, 10.8142, 9.4015) in component "Connection"
fillet "Fillet1" radius 0.25 5 edges at (0, 0, 5.5) (0, 1.65, 0) (4.5, 0, 0) (9, 1.65, 0) (9, 0, 5.5) on bodies 10 in component "DC Jack"
chamfer "Chamfer1''''''''''''" distance 0.25 angle 45 1 edges at (5.6753, 0, 7.7801) on bodies 10 in component "DC Jack"
fillet "Fillet1'" radius 1 1 edges at (3.3346, 1.5, 4.298) on bodies 11 in component "Connection"
sketch "Sketch3 (3)" plane through (0, 0, 0) normal (-1, 0, 0) x (0, 0, 1) in component "Connection"
  line L0 (0.25, 3.3) -> (0.25, 0.25)
  line L1 (0.25, 0.25) -> (11, 0.25)
  line L2 (11, 0.25) -> (11, 11.8)
  line L3 (11, 11.8) -> (4.75, 11.8)
  line L4 (4.75, 11.8) -> (4.75, 3.3)
  line L5 (4.75, 3.3) -> (0.25, 3.3)
  line L6 (4.75, 11.8) -> (12.85, 11.8)
  line L7 (12.85, 11.8) -> (12.85, 9.7)
  line L8 (12.85, 9.7) -> (4.75, 9.7)
  line L9 (4.75, 9.7) -> (4.75, 11.8)
  dimension "d24_5" = 2.1
  dimension "d25_5" = 8.1
extrude "Extrude3'" add sketch "Sketch3 (3)" along normal blind 0.6 separate body contours L2 L3 L4 L6 L8 L9 | L2 L6 L7 L8 makes body 13 in component "Connection"
sketch "Sketch4 (2)" plane through (0, 14.2, 0) normal (0, 1, 0) x (-1, 0, 0) in component "Connection"
  line L0 (-0.55, 4.75) -> (-0.55, 11)
  line L1 (-0.55, 11) -> (-8.45, 11)
  line L2 (-8.45, 11) -> (-8.45, 4.75)
  arc A0 (-8.45, 4.75) -> (-0.55, 4.75) centre (-4.5, 4.75) ccw
  line L3 (-3.25, 3.5) -> (-5.75, 3.5)
  line L4 (-5.75, 3.5) -> (-5.75, 12.8738)
  line L5 (-5.75, 12.8738) -> (-3.25, 12.8738)
  line L6 (-3.25, 12.8738) -> (-3.25, 3.5)
  circle A1 centre (-4.5, 4.75) radius 1.25
extrude "Extrude4" add sketch "Sketch4 (2)" along normal blind 0.6 separate body contours L1 L4 L6 A1 | L1 L4 L5 L6 | A1 | L3 L6 A1 | L3 L4 A1 makes body 14 in component "Connection"
sketch "Sketch5" plane through (0, 0, 11) normal (0, 0, 1) x (1, 0, 0) in component "Connection"
  arc A0 (8.75, 0) -> (9, 0.25) centre (8.75, 0.25) ccw
  line L0 (9, 0.25) -> (9, 11.8)
  line L1 (9, 11.8) -> (8.45, 11.8)
  line L2 (8.45, 11.8) -> (8.45, 14.2)
  line L3 (8.45, 14.2) -> (0.55, 14.2)
  line L4 (0.55, 14.2) -> (0.55, 11.8)
  line L5 (0.55, 11.8) -> (0, 11.8)
  line L6 (0, 11.8) -> (0, 0.25)
  arc A1 (0, 0.25) -> (0.25, 0) centre (0.25, 0.25) ccw
  line L7 (0.25, 0) -> (8.75, 0)
  line L8 (4.5, 14.2) -> (4.5, 9.8) construction
  line L9 (3.45, 9.8) -> (5.55, 9.8)
  line L10 (5.55, 9.8) -> (5.55, 9.2)
  line L11 (5.55, 9.2) -> (3.45, 9.2)
  line L12 (3.45, 9.2) -> (3.45, 9.8)
  dimension "d30_1" = 4.4
  dimension "d31_1" = 2.1
  dimension "d32_1" = 0.6
extrude "Extrude5" add sketch "Sketch5" along normal up to surface (1.8738 mm away) separate body contours L9 L10 L11 L12 makes body 15 in component "Connection"
sketch "Sketch2 (4)" plane through (0, -0.073, 0) normal (0, 1, 0) x (-1, 0, 0) in component "Arduino Leonardo"
  circle A0 centre (13.3359, 12.975) radius 0.3175
  circle A1 centre (13.3359, 17.825) radius 0.3175
  circle A2 centre (-4.4644, 3.0194) radius 0.3175
  circle A3 centre (-9.5443, 2.9966) radius 0.3175
  circle A4 centre (-14.6243, 2.9739) radius 0.3175
  circle A5 centre (-19.7042, 2.9511) radius 0.3175
  circle A6 centre (-24.7842, 2.9284) radius 0.3175
  circle A7 centre (-31.1241, 2.9) radius 0.3175
  circle A8 centre (-36.2041, 2.9) radius 0.3175
  circle A9 centre (-41.2841, 2.9) radius 0.3175
  circle A10 centre (-46.3641, 2.9) radius 0.3175
  circle A11 centre (-48.8641, 38.4601) radius 0.3175
  circle A12 centre (-46.3241, 35.9201) radius 0.3175
  circle A13 centre (-46.3241, 41.0001) radius 0.3175
  circle A14 centre (-13.4241, 51.5) radius 0.3175
  circle A15 centre (-18.5041, 51.5) radius 0.3175
  circle A16 centre (-23.5841, 51.5) radius 0.3175
  circle A17 centre (-28.6641, 51.5) radius 0.3175
  circle A18 centre (-36.2041, 51.5) radius 0.3175
  circle A19 centre (-41.2841, 51.5) radius 0.3175
  circle A20 centre (-46.3641, 51.5) radius 0.3175
  circle A21 centre (-43.8241, 51.5) radius 0.3175
  circle A22 centre (-38.7441, 51.5) radius 0.3175
  circle A23 centre (-33.6641, 51.5) radius 0.3175
  circle A24 centre (-26.1241, 51.5) radius 0.3175
  circle A25 centre (-21.0441, 51.5) radius 0.3175
  circle A26 centre (-15.9641, 51.5) radius 0.3175
  circle A27 centre (-10.8841, 51.5) radius 0.3175
  circle A28 centre (-46.3241, 38.4601) radius 0.3175
  circle A29 centre (-48.8641, 35.9201) radius 0.3175
  circle A30 centre (-48.8641, 41.0001) radius 0.3175
  circle A31 centre (-43.8241, 2.9) radius 0.3175
  circle A32 centre (-38.7441, 2.9) radius 0.3175
  circle A33 centre (-33.6641, 2.9) radius 0.3175
  circle A34 centre (-28.5841, 2.9114) radius 0.3175
  circle A35 centre (-22.2442, 2.9398) radius 0.3175
  circle A36 centre (-17.1643, 2.9625) radius 0.3175
  circle A37 centre (-12.0843, 2.9853) radius 0.3175
  circle A38 centre (-7.0044, 3.008) radius 0.3175
  circle A39 centre (-1.9244, 3.0307) radius 0.3175
  circle A40 centre (-48.6141, 46.05) radius 1.75
  circle A41 centre (1.8359, 3.15) radius 1.75
  circle A42 centre (3.3359, 51.25) radius 1.75
  circle A43 centre (-48.6141, 18.55) radius 1.75
  line L0 (-48.8641, 51.2) -> (-51.3641, 48.7)
  line L1 (-51.3641, 48.7) -> (-51.3641, 15.9)
  line L2 (-51.3641, 15.9) -> (-48.8641, 13.4)
  line L3 (-48.8641, 13.4) -> (-48.8641, 2.0476)
  line L4 (-48.8641, 2.0476) -> (-47.2166, 0.4)
  line L5 (-47.2166, 0.4) -> (17.3359, 0.4)
  line L6 (17.3359, 0.4) -> (17.3359, 54)
  line L7 (17.3359, 54) -> (-48.8641, 54)
  line L8 (-48.8641, 54) -> (-48.8641, 51.2)
  line L9 (12, 12) -> (19, 12)
  line L10 (19, 12) -> (19, 19)
  line L11 (19, 19) -> (12, 19)
  line L12 (12, 19) -> (12, 12)
extrude "Extrude1'''''''''''''''" add sketch "Sketch2 (4)" along normal blind 2.5 separate body contours A0 | A1 | L6 L9 L10 L11 | L6 L9 L11 L12 makes body 16 in component "MicroUSBMockup"
component "Arduino Leonardo" placed x (1, 0, 0) y (0, 1, 0) z (0, 0, 1) at (17.3359, 1.693, -0.4)
component "PCB" placed x (1, 0, 0) y (0, 1, 0) z (0, 0, 1) at (-17.3359, -1.693, 0.4) in component "Arduino Leonardo"
component "DC Jack v3" placed x (0, 0, -1) y (0, 1, 0) z (1, 0, 0) at (-36.3359, -1.693, 50.4) in component "Arduino Leonardo"
component "MicroUSBMockup" placed x (1, 0, 0) y (0, 1, 0) z (0, 0, 1) at (0, 0, 0) in component "Arduino Leonardo"
component "Pins straight female v5" placed x (0, 1, 0) y (-1, 0, 0) z (0, 0, 1) at (64.0175, -1.555, 50.7825) in component "PCB"
component "Pins straight female v6" placed x (0, 1, 0) y (-1, 0, 0) z (0, 0, 1) at (46.3175, -1.555, 50.7825) in component "PCB"
component "Pins straight female v6" placed x (0, 1, 0) y (-1, 0, 0) z (0, 0, 1) at (64.0175, -1.555, 2.1825) in component "PCB"
component "Pins straight female v7" placed x (0, 1, 0) y (-1, 0, 0) z (0, 0, 1) at (42.4376, -1.555, 2.2109) in component "PCB"
component "Pins straight female v8" placed x (0, 1, 0) y (0, 0, 1) z (1, 0, 0) at (63.3425, -1.555, 35.2026) in component "PCB"
component "Pins straight female v8" placed x (0, 1, 0) y (0, 0, 1) z (1, 0, 0) at (65.8825, -1.555, 35.2026) in component "PCB"
component "Header" placed x (1, 0, 0) y (0, 1, 0) z (0, 0, 1) at (0, 0, 0) in component "Pins straight female v5"
component "Header" placed x (1, 0, 0) y (0, 1, 0) z (0, 0, 1) at (0, 2.54, 0) in component "Pins straight female v5"
component "Header" placed x (1, 0, 0) y (0, 1, 0) z (0, 0, 1) at (0, 5.08, 0) in component "Pins straight female v5"
component "Header" placed x (1, 0, 0) y (0, 1, 0) z (0, 0, 1) at (0, 7.62, 0) in component "Pins straight female v5"
component "Header" placed x (1, 0, 0) y (0, 1, 0) z (0, 0, 1) at (0, 10.16, 0) in component "Pins straight female v5"
component "Header" placed x (1, 0, 0) y (0, 1, 0) z (0, 0, 1) at (0, 12.7, 0) in component "Pins straight female v5"
component "Pin" placed x (1, 0, 0) y (0, 1, 0) z (0, 0, 1) at (0, 0, 0) in component "Header"
component "Plastic" placed x (1, 0, 0) y (0, 1, 0) z (0, 0, 1) at (0, 0, 0) in component "Header"
component "Header (1)" placed x (1, 0, 0) y (0, 1, 0) z (0, 0, 1) at (0, 0, 0) in component "Pins straight female v6"
component "Header (1)" placed x (1, 0, 0) y (0, 1, 0) z (0, 0, 1) at (0, 2.54, 0) in component "Pins straight female v6"
component "Header (1)" placed x (1, 0, 0) y (0, 1, 0) z (0, 0, 1) at (0, 5.08, 0) in component "Pins straight female v6"
component "Header (1)" placed x (1, 0, 0) y (0, 1, 0) z (0, 0, 1) at (0, 7.62, 0) in component "Pins straight female v6"
component "Header (1)" placed x (1, 0, 0) y (0, 1, 0) z (0, 0, 1) at (0, 10.16, 0) in component "Pins straight female v6"
component "Header (1)" placed x (1, 0, 0) y (0, 1, 0) z (0, 0, 1) at (0, 12.7, 0) in component "Pins straight female v6"
component "Header (1)" placed x (1, 0, 0) y (0, 1, 0) z (0, 0, 1) at (0, 15.24, 0) in component "Pins straight female v6"
component "Header (1)" placed x (1, 0, 0) y (0, 1, 0) z (0, 0, 1) at (0, 17.78, 0) in component "Pins straight female v6"
component "Pin (1)" placed x (1, 0, 0) y (0, 1, 0) z (0, 0, 1) at (0, 0, 0) in component "Header (1)"
component "Plastic (1)" placed x (1, 0, 0) y (0, 1, 0) z (0, 0, 1) at (0, 0, 0) in component "Header (1)"
component "Header (2)" placed x (1, 0, 0) y (0, 1, 0) z (0, 0, 1) at (0, 0, 0) in component "Pins straight female v7"
component "Header (2)" placed x (1, 0, 0) y (0, 1, 0) z (0, 0, 1) at (0, 2.54, 0) in component "Pins straight female v7"
component "Header (2)" placed x (1, 0, 0) y (0, 1, 0) z (0, 0, 1) at (0, 5.08, 0) in component "Pins straight female v7"
component "Header (2)" placed x (1, 0, 0) y (0, 1, 0) z (0, 0, 1) at (0, 7.62, 0) in component "Pins straight female v7"
component "Header (2)" placed x (1, 0, 0) y (0, 1, 0) z (0, 0, 1) at (0, 10.16, 0) in component "Pins straight female v7"
component "Header (2)" placed x (1, 0, 0) y (0, 1, 0) z (0, 0, 1) at (0, 12.7, 0) in component "Pins straight female v7"
component "Header (2)" placed x (1, 0, 0) y (0, 1, 0) z (0, 0, 1) at (0, 15.24, 0) in component "Pins straight female v7"
component "Header (2)" placed x (1, 0, 0) y (0, 1, 0) z (0, 0, 1) at (0, 17.78, 0) in component "Pins straight female v7"
component "Header (2)" placed x (1, 0, 0) y (0, 1, 0) z (0, 0, 1) at (0, 20.32, 0) in component "Pins straight female v7"
component "Header (2)" placed x (1, 0, 0) y (0, 1, 0) z (0, 0, 1) at (0, 22.86, 0) in component "Pins straight female v7"
component "Pin (2)" placed x (1, 0, 0) y (0, 1, 0) z (0, 0, 1) at (0, 0, 0) in component "Header (2)"
component "Plastic (2)" placed x (1, 0, 0) y (0, 1, 0) z (0, 0, 1) at (0, 0, 0) in component "Header (2)"
component "Header (3)" placed x (1, 0, 0) y (0, 1, 0) z (0, 0, 1) at (0, 0, 0) in component "Pins straight female v8"
component "Header (3)" placed x (1, 0, 0) y (0, 1, 0) z (0, 0, 1) at (0, 2.54, 0) in component "Pins straight female v8"
component "Header (3)" placed x (1, 0, 0) y (0, 1, 0) z (0, 0, 1) at (0, 5.08, 0) in component "Pins straight female v8"
component "Pin (3)" placed x (1, 0, 0) y (0, 1, 0) z (0, 0, 1) at (0, 0, 0) in component "Header (3)"
component "Plastic (3)" placed x (1, 0, 0) y (0, 1, 0) z (0, 0, 1) at (0, 0, 0) in component "Header (3)"
component "DC Jack" placed x (1, 0, 0) y (0, 0, 1) z (0, -1, 0) at (0.4, 12.6198, 16.5) in component "DC Jack v3"
component "Connection" placed x (1, 0, 0) y (0, 1, 0) z (0, 0, 1) at (0, 0, 0) in component "DC Jack"
equation "d14 = ( 3.5 / 2 ) * 1 mm"
equation "d17 = ( 3.5 / 2 ) * 1 mm"
equation "d18 = ( 3.5 / 2 ) * 1 mm"
equation "pinCount = 6"
equation "d12_1 = plasticHeight"
equation "d13_1 = 0.025 in / 2"
equation "d19_1 = pinCount"
equation "d21_1 = pinCount"
equation "plasticHeight = 0.34 in"
equation "pinCount_1 = 8"
equation "d12_2 = plasticHeight_1"
equation "d13_2 = 0.025 in / 2"
equation "d19_2 = pinCount_1"
equation "d21_2 = pinCount_1"
equation "plasticHeight_1 = 0.34 in"
equation "pinCount_2 = 10"
equation "d12_3 = plasticHeight_2"
equation "d13_3 = 0.025 in / 2"
equation "d19_3 = pinCount_2"
equation "d21_3 = pinCount_2"
equation "plasticHeight_2 = 0.34 in"
equation "pinCount_3 = 3"
equation "d12_4 = plasticHeight_3"
equation "d13_4 = 0.025 in / 2"
equation "d19_4 = pinCount_3"
equation "d21_4 = pinCount_3"
equation "plasticHeight_3 = 0.34 in"
equation "d15_5 = 9.60 mm - 1.5 mm"
equation "d19_5 = -2.27 mm * 2"
